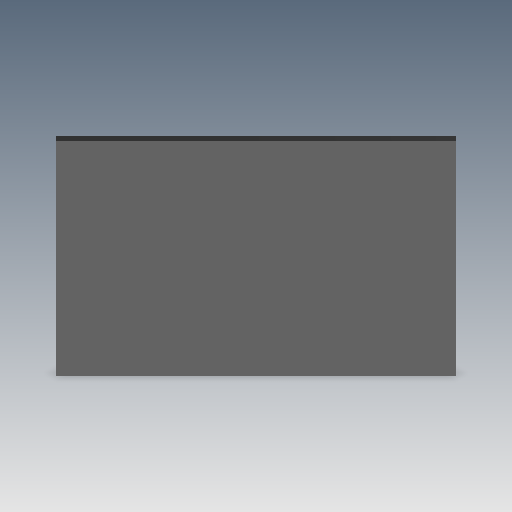
# Autodesk Inventor part: BeamsplitterReflect
Saved by Autodesk Inventor 2026 (Build 300175050, 175E)
## iProperties
Created: 2025-08-02
Part Number: BeamsplitterReflect
Material: Generic
Document SubType Name: Modeling
Designer: aman0
Density: 1 g/cm^3
Appearance: Default
Author: aman0
Autodesk Inventor part; units mm, degrees
ref_plane "YZ Plane" through (0, 0, 0) normal (1, 0, 0) x (0, 1, 0)
ref_plane "XZ Plane" through (0, 0, 0) normal (0, 1, 0) x (-1, 0, 0)
ref_plane "XY Plane" through (0, 0, 0) normal (0, 0, 1) x (1, 0, 0)
sketch "Sketch1" plane through (0, 0, 0) normal (0, 1, 0) x (-1, 0, 0)
  line L0 (12.5, 12.5) -> (12.5, -12.5)
  line L1 (12.5, -12.5) -> (-12.5, -12.5)
  line L2 (-12.5, -12.5) -> (-12.5, 12.5)
  line L3 (-12.5, 12.5) -> (12.5, 12.5)
  line L4 (12.5, 12.5) -> (-12.5, -12.5) construction
  line L5 (12.5, -12.5) -> (-12.5, 12.5) construction
  line L6 (-12, -12.5) -> (12.5, 12)
  line L7 (12.5, 12) -> (12, 12.5)
  line L8 (12, 12.5) -> (-12.5, -12)
  line L9 (-12.5, -12) -> (-12, -12.5)
  point P0 (0, 0)
  dimension "d0" = 25
  dimension "d1" = 25
  dimension "d2" = 0.5
  constraints: 20 end point, 4 parallel, 4 point on line, 2 midpoint, 2 perpendicular, 1 vertical
  measures "d0" distance of L0.start L0.end
  measures "d1" distance of L0.end L1.end
  measures "d2" distance of L0.start L6.end
extrude "Extrusion1" add sketch "Sketch1" along normal mid plane 25 contours L6 L9 L8 L7
body "Solid1"
